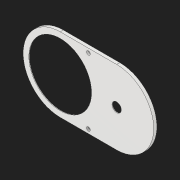
# Autodesk Inventor part: HA013
Saved by Autodesk Inventor 2017 SP1 (Build 210196100, 196)
## iProperties
Created: 2018-02-26
Part Number: HA013
Material: ABS Plastic
Document SubType Name: Modeling
Designer: Zach
Density: 1.06 g/cm^3
Appearance: CR White
Author: Zach
Autodesk Inventor part; units mm, degrees
ref_plane "YZ Plane" through (0, 0, 0) normal (1, 0, 0) x (0, 1, 0)
ref_plane "XZ Plane" through (0, 0, 0) normal (0, 1, 0) x (-1, 0, 0)
ref_plane "XY Plane" through (0, 0, 0) normal (0, 0, 1) x (1, 0, 0)
sketch "Sketch1" plane through (0, 0, 0) normal (0, 0, 1) x (1, 0, 0)
  circle A0 centre (0, 0) radius 59
  circle A1 centre (90, 0) radius 59
  line L0 (0, 59) -> (90, 59)
  line L1 (90, -59) -> (0, -59)
  dimension "d0" = 118
  dimension "d1" = 118
  dimension "d2" = 90
  constraints: 4 end point, 4 point on circle, 4 tangent, 2 centre point, 1 coincident, 1 horizontal alignment
  measures "d0" diameter of A0
  measures "d1" diameter of A1
  measures "d2" distance of A1.centre point (0, 0)
extrude "Extrusion1" add sketch "Sketch1" along normal blind 5
sketch "Sketch2" plane through (0, 0, 0) normal (0, 0, -1) x (-1, 0, 0)
  arc A0 (0, -59) -> (0, 59) centre (0, 0) ccw projected
  line L0 (-90, 59) -> (0, 59) projected
  arc A1 (-90, 59) -> (-90, -59) centre (-90, 0) ccw projected
  line L1 (0, -59) -> (-90, -59) projected
  arc A2 (0, -56) -> (0, 56) centre (0, 0) ccw
  line L2 (0, -56) -> (-90, -56)
  arc A3 (-90, 56) -> (-90, -56) centre (-90, 0) ccw
  line L3 (-90, 56) -> (0, 56)
  dimension "d5" = 3
  constraints: 4 end point, 4 point on circle, 2 centre point, 3 other
  measures "d5" radial gap between concentric circles of A0 A2
extrude "Extrusion2" cut sketch "Sketch2" against normal blind 4 contours L2 A3 L3 A2
sketch "Sketch3" plane through (0, 0, 5) normal (0, 0, 1) x (1, 0, 0)
  circle A0 centre (90, 0) radius 7.5
  arc A1 (90, -59) -> (90, 59) centre (90, 0) ccw projected
  circle A2 centre (0, 0) radius 50
  dimension "d8" = 15
  dimension "d9" = 100
  constraints: 2 centre point, 2 coincident
  measures "d8" diameter of A0
  measures "d9" diameter of A2
extrude "Extrusion3" cut sketch "Sketch3" against normal through all
sketch "Sketch4" plane through (0, 0, 5) normal (0, 0, 1) x (1, 0, 0)
  line L0 (45, 52.5) -> (45, -52.5) construction
  line L1 (90, 59) -> (0, 59) construction
  circle A0 centre (45, 52.5) radius 1.5
  circle A1 centre (45, -52.5) radius 1.5
  point P0 (0, 0)
  point P1 (45, 0)
  point P2 (45, 59)
  dimension "d12" = 105
  dimension "d13" = 3
  dimension "d14" = 3
  constraints: 2 centre point, 2 coincident, 2 end point, 2 midpoint, 1 horizontal alignment, 1 vertical, 1 vertical alignment
  measures "d12" distance of L0.start L0.end
  measures "d13" diameter of A0
  measures "d14" diameter of A1
extrude "Extrusion4" cut sketch "Sketch4" against normal through all
sketch "Sketch5" plane through (0, 0, 4) normal (0, 0, -1) x (-1, 0, 0)
  circle A0 centre (-45, -52.5) radius 1.5 projected
  circle A1 centre (-45, 52.5) radius 1.5 projected
  circle A2 centre (-45, 52.5) radius 6.5
  line L0 (-38.5, 52.5) -> (-38.5, 59)
  line L1 (-51.5, 52.5) -> (-51.5, 59)
  line L2 (-90, 59) -> (0, 59) projected
  line L3 (-38.5, 59) -> (-51.5, 59)
  line L4 (-51.5, 59) -> (-38.5, 59)
  circle A3 centre (-45, -52.5) radius 6.5
  line L5 (-38.5, -52.5) -> (-38.5, -59)
  line L6 (0, -59) -> (-90, -59) projected
  line L7 (-38.5, -59) -> (-51.5, -59)
  line L8 (-51.5, -59) -> (-51.5, -52.5)
  point P0 (0, 0)
  dimension "d17" = 13
  dimension "d18" = 13
  constraints: 14 end point, 4 point on circle, 4 tangent, 4 vertical, 3 point on line, 2 centre point, 2 coincident, 1 collinear
  measures "d17" diameter of A2
  measures "d18" diameter of A3
extrude "Extrusion5" add sketch "Sketch5" along normal blind 4
sketch "Sketch6" plane through (0, 0, 5) normal (0, 0, 1) x (1, 0, 0)
  circle A0 centre (45, -52.5) radius 1.5 projected
  circle A1 centre (45, 52.5) radius 1.5 projected
  circle A2 centre (45, 52.5) radius 1.5 projected
  circle A3 centre (45, 52.5) radius 3
  circle A4 centre (45, -52.5) radius 3
  point P0 (0, 0)
  dimension "d21" = 6
  dimension "d22" = 6
  constraints: 2 centre point, 2 coincident
  measures "d21" diameter of A3
  measures "d22" diameter of A4
extrude "Extrusion6" cut sketch "Sketch6" against normal blind 3 contours A0 | A1 | A3 | A4
body "Solid1"
